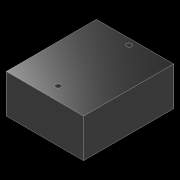
# Autodesk Inventor part: EscMockup
Saved by Autodesk Inventor 2021 (Build 250183000, 183)
## iProperties
Created: 2021-03-28
Part Number: EscMockup
Material: Generic
Document SubType Name: Modeling
Designer: Esketitttttt
Density: 2.46044 g/cm^3
Appearance: Glossy - Black
Mass: 544.311 g
Surface Area: 232.258 cm^2
Volume: 221.225 cm^3
Author: Esketitttttt
Autodesk Inventor part; units mm, degrees
ref_plane "YZ Plane" through (0, 0, 0) normal (1, 0, 0) x (0, 1, 0)
ref_plane "XZ Plane" through (0, 0, 0) normal (0, 1, 0) x (-1, 0, 0)
ref_plane "XY Plane" through (0, 0, 0) normal (0, 0, 1) x (1, 0, 0)
sketch "Sketch1" plane through (0, 0, 0) normal (0, 1, 0) x (-1, 0, 0)
  line L0 (0, 0) -> (76.2, 0)
  line L1 (76.2, 0) -> (76.2, -76.2)
  line L2 (76.2, -76.2) -> (0, -76.2)
  line L3 (0, -76.2) -> (0, 0)
  line L4 (38.1, 0) -> (38.1, -6.858) construction
  line L5 (38.1, -6.858) -> (38.1, -76.708) construction
  line L6 (76.2, -76.2) -> (0, -76.2)
  line L7 (0, -76.2) -> (0, -82.55)
  line L8 (0, -82.55) -> (76.2, -82.55)
  line L9 (76.2, -82.55) -> (76.2, -76.2)
  line L10 (76.2, 0) -> (0, 0)
  line L11 (0, 0) -> (0, 6.35)
  line L12 (0, 6.35) -> (76.2, 6.35)
  line L13 (76.2, 6.35) -> (76.2, 0)
  point P0 (0.5337, -76.2)
  point P1 (0.741, 0)
  dimension "d0" = 76.2
  dimension "d1" = 76.2
  dimension "d4" = 6.858
  dimension "d5" = 69.85
  dimension "d8" = 6.35
  dimension "d9" = 6.35
  constraints: 28 end point, 6 parallel, 3 horizontal, 3 perpendicular, 2 coincident, 2 vertical, 1 midpoint
  measures "d0" distance of L1.end L2.end
  measures "d1" distance of L0.end L1.end
  measures "d4" distance of L4.start L4.end
  measures "d5" distance of L4.end L5.end
  measures "d8" distance of L2.end L7.end
  measures "d9" distance of L0.start L11.end
extrude "Extrusion1" add sketch "Sketch1" along normal blind 38.1
hole "Hole1" at (-38.1, 0, -6.858) at (-38.1, 0, -76.708) direction (0, 1, 0) diameter 5.1054 end through all clearance for "Flat Head Machine Screw (82)" size "#10" standard "Ansi Unified Screw Threads"
body "Solid1"
